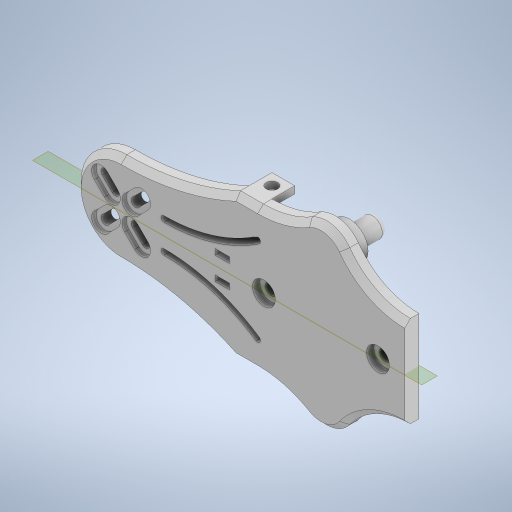
# Autodesk Inventor part: BLDC_Arm_2
Saved by Autodesk Inventor 2024 (Build 280153000, 153)
## iProperties
Created: 2024-04-12
Part Number: BLDC_Arm_2
Material: Generic
Document SubType Name: Modeling
Designer: CJ110
Density: 1 g/cm^3
Appearance: Default
Author: CJ110
Autodesk Inventor part; units mm, degrees
ref_plane "YZ Plane" through (0, 0, 0) normal (1, 0, 0) x (0, 1, 0)
ref_plane "XZ Plane" through (0, 0, 0) normal (0, 1, 0) x (-1, 0, 0)
ref_plane "XY Plane" through (0, 0, 0) normal (0, 0, 1) x (1, 0, 0)
sketch "Sketch1" plane through (0, 0, 0) normal (0, 0, 1) x (1, 0, 0)
  arc A0 (0, 16) -> (0, -16) centre (0, 0) ccw
  line L0 (0, 16) -> (99.4033, 16)
  line L1 (99.4033, 16) -> (99.4033, -16)
  line L2 (99.4033, -16) -> (0, -16)
  line L3 (0, -16) -> (0, 16) construction
  line L4 (39.8634, 25) -> (99.4033, 25)
  line L5 (99.4033, 25) -> (99.4033, -25)
  line L6 (99.4033, -25) -> (39.8634, -25)
  line L7 (39.8634, -25) -> (39.8634, 25)
  arc A1 (39.8634, -25) -> (0, -16) centre (0, -108.7828) ccw
  arc A2 (0, 16) -> (39.8634, 25) centre (0, 108.7828) ccw
  circle A3 centre (50.0625, 0) radius 2
  circle A4 centre (90.0625, 0) radius 2
  line L8 (-16, 0) -> (99.4033, 0) construction
  line L9 (-7.0711, 7.0711) -> (-3.5356, 3.5356) construction
  line L10 (-8.1318, 6.0104) -> (-4.5962, 2.4749)
  line L11 (-2.4749, 4.5962) -> (-6.0104, 8.1318)
  arc A5 (-6.0104, 8.1318) -> (-8.1318, 6.0104) centre (-7.0711, 7.0711) ccw
  arc A6 (-4.5962, 2.4749) -> (-2.4749, 4.5962) centre (-3.5356, 3.5356) ccw
  line L12 (0, 0) -> (-8.1318, 8.1318) construction
  arc A7 (-2.4749, -4.5962) -> (-4.5962, -2.4749) centre (-3.5356, -3.5356) ccw
  line L13 (-4.5962, -2.4749) -> (-8.1318, -6.0104)
  arc A8 (-8.1318, -6.0104) -> (-6.0104, -8.1318) centre (-7.0711, -7.0711) ccw
  line L14 (-6.0104, -8.1318) -> (-2.4749, -4.5962)
  arc A9 (4.5962, -2.4749) -> (2.4749, -4.5962) centre (3.5356, -3.5356) ccw
  line L15 (2.4749, -4.5962) -> (6.0104, -8.1318)
  arc A10 (6.0104, -8.1318) -> (8.1318, -6.0104) centre (7.0711, -7.0711) ccw
  line L16 (8.1318, -6.0104) -> (4.5962, -2.4749)
  arc A11 (2.4749, 4.5962) -> (4.5962, 2.4749) centre (3.5356, 3.5356) ccw
  line L17 (4.5962, 2.4749) -> (8.1318, 6.0104)
  arc A12 (8.1318, 6.0104) -> (6.0104, 8.1318) centre (7.0711, 7.0711) ccw
  line L18 (6.0104, 8.1318) -> (2.4749, 4.5962)
  point P0 (39.8634, 0)
  point P1 (99.4033, -16)
  point P2 (99.4033, 16)
  point P3 (-5.3033, 5.3033)
  point P4 (-2.4749, 2.4749)
  point P5 (-2.4749, -2.4749)
  point P6 (-8.1318, -8.1318)
  point P7 (2.4749, -2.4749)
  point P8 (8.1318, -8.1318)
  point P9 (2.4749, 2.4749)
  point P10 (8.1318, 8.1318)
  dimension "d3" = 50
  dimension "d4" = 59.5399
  dimension "d12" = 4
  dimension "d13" = 40
  dimension "d15" = 9.3408
  dimension "d44" = 16
  dimension "d45" = 99.4033
  dimension "d46" = 3
  dimension "d47" = 8
  dimension "d48" = 45
  dimension "d49" = 2.4749
  dimension "d52" = 360
  constraints: 40 end point, 25 point on circle, 13 centre point, 7 tangent, 5 parallel, 4 midpoint, 3 horizontal, 2 collinear, 2 perpendicular, 2 point on line, 1 coincident, 1 equal radius, 1 horizontal alignment, 49 other
  measures "d3" distance between parallel lines of L6 L4
  measures "d4" distance between parallel lines of L5 L7
  measures "d12" diameter of A4
  measures "d13" distance of A3.centre A4.centre
  measures "d15" distance from line of L1 A4.centre
  measures "d44" radius of A0
  measures "d45" distance from line of point (0, 0) L5
  measures "d46" distance between parallel lines of L10 L11
  measures "d47" distance of point (-2.475, 2.475) L12.end
  measures "d48" angle of L8 L12
  measures "d49" distance from line of L8 point (-2.475, 2.475)
extrude "Extrusion1" add sketch "Sketch1" along normal blind 5
ref_plane "Work Plane1" through (39.8634, 0, 0) normal (0, -1, 0) x (1, 0, 0)
sketch "Sketch4" plane through (0, 0, 5) normal (0, 0, 1) x (1, 0, 0)
  arc A0 (15, 6) -> (47.3064, 15.8305) centre (15, 64.0002) ccw
  arc A1 (15, 4) -> (48.4204, 14.1695) centre (15, 64.0002) ccw
  circle A2 centre (47.8634, 15) radius 1
  circle A3 centre (15, 5) radius 1
  arc A4 (0, 16) -> (39.8634, 25) centre (0, 108.7828) ccw projected
  line L0 (99.4033, 25) -> (39.8634, 25) projected
  line L1 (122.484, 0) -> (-39.0807, 0) projected
  line L2 (15, 4) -> (47.8634, 4) construction
  point P0 (0, 0)
  dimension "d16" = 2
  dimension "d17" = 10
  dimension "d18" = 8
  dimension "d19" = 15
  dimension "d20" = 5
  constraints: 8 point on circle, 5 tangent, 4 centre point, 2 end point, 1 concentric, 1 equal radius, 1 horizontal, 1 vertical alignment
  measures "d16" diameter of A2
  measures "d17" distance from line of L0 A2.centre
  measures "d18" horizontal distance of L0.end A2.centre
  measures "d19" horizontal distance of point (0, 0) A3.centre
  measures "d20" distance from line of L1 A3.centre
extrude "Extrusion3" cut sketch "Sketch4" against normal through all
mirror "Mirror1" about plane through (39.8634, 0, 0) normal (0, -1, 0) of "Extrusion3"
sketch "Sketch5" plane through (0, 0, 0) normal (0, 0, -1) x (-1, 0, 0)
  arc A0 (-15, -4) -> (-48.4204, -14.1695) centre (-15, -64.0002) ccw projected
  arc A1 (-15, -6) -> (-15, -4) centre (-15, -5) ccw projected
  arc A2 (-15, -6) -> (-47.3064, -15.8305) centre (-15, -64.0002) ccw projected
  arc A3 (-48.4204, -14.1695) -> (-47.3064, -15.8305) centre (-47.8634, -15) ccw projected
  arc A4 (-47.3064, 15.8305) -> (-15, 6) centre (-15, 64.0002) ccw projected
  arc A5 (-15, 4) -> (-15, 6) centre (-15, 5) ccw projected
  arc A6 (-48.4204, 14.1695) -> (-15, 4) centre (-15, 64.0002) ccw projected
  arc A7 (-47.3064, 15.8305) -> (-48.4204, 14.1695) centre (-47.8634, 15) ccw projected
  arc A8 (0, -16) -> (0, 16) centre (0, 0) ccw projected
  arc A9 (-39.8634, 25) -> (0, 16) centre (0, 108.7828) ccw projected
  line L0 (-99.4033, 25) -> (-39.8634, 25) projected
  line L1 (-99.4033, -25) -> (-99.4033, 25) projected
  line L2 (-39.8634, -25) -> (-99.4033, -25) projected
  arc A10 (0, -16) -> (-39.8634, -25) centre (0, -108.7828) ccw projected
  circle A11 centre (-50.0625, 0) radius 2 projected
  circle A12 centre (-90.0625, 0) radius 2 projected
  line L3 (-39.8634, 25) -> (-47.8634, 25)
  line L4 (-47.8634, 25) -> (-47.8634, 22.5)
  line L5 (-47.8634, 22.5) -> (-39.8634, 22.5)
  line L6 (-39.8634, 22.5) -> (-39.8634, 25)
  dimension "d23" = 8
  dimension "d24" = 2.5
  constraints: 8 end point, 2 parallel, 1 horizontal, 1 perpendicular
  measures "d23" distance of L4.end L5.end
  measures "d24" distance of L3.end L4.end
extrude "Extrusion4" add sketch "Sketch5" along normal blind 8 contours L6 L5 L4 L0
sketch "Sketch6" plane through (39.8634, 25, 5) normal (0, 1, 0) x (1, 0, 0)
  line L0 (59.5399, 5) -> (8, 5) projected
  line L1 (8, 5) -> (8, 13) projected
  line L2 (0, 13) -> (8, 13) projected
  line L3 (0, 5) -> (0, 13) projected
  line L4 (0, 5) -> (0, 0) projected
  line L5 (59.5399, 0) -> (0, 0) projected
  line L6 (59.5399, 5) -> (59.5399, 0) projected
  circle A0 centre (4, 9) radius 2
  line L7 (4, 13) -> (4, 9) construction
  point P0 (-39.8634, 5)
  dimension "d27" = 4
  dimension "d28" = 4
  constraints: 2 end point, 1 centre point, 1 midpoint, 1 vertical
  measures "d27" distance from line of L2 L7.end
  measures "d28" diameter of A0
extrude "Extrusion5" cut sketch "Sketch6" against normal up to next contours A0
mirror "Mirror2" about plane through (39.8634, 0, 0) normal (0, -1, 0) of "Extrusion4", "Extrusion5"
sketch "Sketch7" plane through (0, 0, 0) normal (0, 0, -1) x (-1, 0, 0)
  circle A0 centre (-90.0625, 0) radius 2 projected
  circle A1 centre (-50.0625, 0) radius 2 projected
  arc A2 (-47.3064, 15.8305) -> (-15, 6) centre (-15, 64.0002) ccw projected
  arc A3 (-15, 4) -> (-15, 6) centre (-15, 5) ccw projected
  arc A4 (-48.4204, 14.1695) -> (-15, 4) centre (-15, 64.0002) ccw projected
  arc A5 (-47.3064, 15.8305) -> (-48.4204, 14.1695) centre (-47.8634, 15) ccw projected
  arc A6 (-15, -4) -> (-48.4204, -14.1695) centre (-15, -64.0002) ccw projected
  arc A7 (-15, -6) -> (-15, -4) centre (-15, -5) ccw projected
  arc A8 (-15, -6) -> (-47.3064, -15.8305) centre (-15, -64.0002) ccw projected
  arc A9 (-48.4204, -14.1695) -> (-47.3064, -15.8305) centre (-47.8634, -15) ccw projected
  line L0 (-47.8634, -25) -> (-47.8634, -22.5) projected
  line L1 (-47.8634, -22.5) -> (-39.8634, -22.5) projected
  line L2 (-39.8634, -22.5) -> (-39.8634, -25) projected
  arc A10 (0, -16) -> (-39.8634, -25) centre (0, -108.7828) ccw projected
  arc A11 (0, -16) -> (0, 16) centre (0, 0) ccw projected
  arc A12 (-39.8634, 25) -> (0, 16) centre (0, 108.7828) ccw projected
  line L3 (-39.8634, 25) -> (-39.8634, 22.5) projected
  line L4 (-39.8634, 22.5) -> (-47.8634, 22.5) projected
  line L5 (-47.8634, 22.5) -> (-47.8634, 25) projected
  line L6 (-99.4033, 25) -> (-47.8634, 25) projected
  line L7 (-99.4033, -25) -> (-99.4033, 25) projected
  line L8 (-47.8634, -25) -> (-99.4033, -25) projected
  circle A13 centre (-70.0625, 21) radius 10
  arc A14 (-65.0249, 29.6384) -> (-47.8634, 25) centre (-47.8634, 59.0667) ccw
  line L9 (-99.4033, 25) -> (-47.8634, 25) projected
  line L10 (39.0807, 0) -> (-122.484, 0) projected
  line L11 (-70.0625, -25) -> (-70.0625, 21) construction
  line L12 (-90.0625, 0) -> (-50.0625, 0) construction
  line L13 (0, 16) -> (-99.4033, 16) construction
  arc A15 (-99.4033, 16) -> (-78.1686, 26.8559) centre (-99.4033, 42.1961) ccw
  point P0 (-92.2616, 25)
  point P1 (-75.1001, 29.6384)
  point P2 (-70.0625, 0)
  point P3 (-60.8973, 25)
  point P4 (-79.2277, 25)
  point P5 (-79.6415, 25)
  dimension "d31" = 20
  dimension "d32" = 21
  constraints: 7 point on circle, 6 end point, 5 tangent, 4 point on line, 3 centre point, 2 perpendicular, 1 coincident, 1 collinear, 1 midpoint, 1 vertical
  measures "d31" diameter of A13
  measures "d32" distance from line of L10 A13.centre
extrude "Extrusion6" add sketch "Sketch7" against normal up to surface (5 mm away) contours A15 A13 L6 | A13 L6 | A13 A14 L6 picked at (-69.5865, 27.6164)
sketch "Sketch8" plane through (0, 0, 0) normal (0, 0, -1) x (-1, 0, 0)
  circle A0 centre (-90.0625, 0) radius 2 projected
  circle A1 centre (-50.0625, 0) radius 2 projected
  arc A2 (-47.3064, 15.8305) -> (-15, 6) centre (-15, 64.0002) ccw projected
  arc A3 (-15, 4) -> (-15, 6) centre (-15, 5) ccw projected
  arc A4 (-48.4204, 14.1695) -> (-15, 4) centre (-15, 64.0002) ccw projected
  arc A5 (-47.3064, 15.8305) -> (-48.4204, 14.1695) centre (-47.8634, 15) ccw projected
  arc A6 (-15, -4) -> (-48.4204, -14.1695) centre (-15, -64.0002) ccw projected
  arc A7 (-15, -6) -> (-15, -4) centre (-15, -5) ccw projected
  arc A8 (-15, -6) -> (-47.3064, -15.8305) centre (-15, -64.0002) ccw projected
  arc A9 (-48.4204, -14.1695) -> (-47.3064, -15.8305) centre (-47.8634, -15) ccw projected
  line L0 (-47.8634, -25) -> (-47.8634, -22.5) projected
  line L1 (-47.8634, -22.5) -> (-39.8634, -22.5) projected
  line L2 (-39.8634, -22.5) -> (-39.8634, -25) projected
  arc A10 (0, -16) -> (-39.8634, -25) centre (0, -108.7828) ccw projected
  arc A11 (0, -16) -> (0, 16) centre (0, 0) ccw projected
  arc A12 (-39.8634, 25) -> (0, 16) centre (0, 108.7828) ccw projected
  line L3 (-39.8634, 25) -> (-39.8634, 22.5) projected
  line L4 (-39.8634, 22.5) -> (-47.8634, 22.5) projected
  line L5 (-47.8634, 22.5) -> (-47.8634, 25) projected
  arc A13 (-65.0249, 29.6384) -> (-47.8634, 25) centre (-47.8634, 59.0667) ccw projected
  arc A14 (-65.0249, 29.6384) -> (-78.1686, 26.8559) centre (-70.0625, 21) ccw projected
  line L6 (-99.4033, 25) -> (-79.6415, 25) projected
  line L7 (-99.4033, -25) -> (-99.4033, 25) projected
  line L8 (-47.8634, -25) -> (-99.4033, -25) projected
  circle A15 centre (-70.0625, 21) radius 6.5
  arc A16 (-79.6415, 25) -> (-78.1686, 26.8559) centre (-99.4033, 42.1961) ccw projected
  dimension "d35" = 13
  constraints: 1 centre point, 1 coincident
  measures "d35" diameter of A15
extrude "Extrusion7" add sketch "Sketch8" along normal blind 5 contours A15
sketch "Sketch9" plane through (70.0625, 21, -5) normal (0, 0, -1) x (-1, 0, 0)
  circle A0 centre (0, 0) radius 3.5
  circle A1 centre (0, 0) radius 6.5 projected
  point P0 (70.0625, -21)
  dimension "d38" = 7
  constraints: 1 centre point, 1 coincident
  measures "d38" diameter of A0
extrude "Extrusion8" add sketch "Sketch9" along normal blind 10 contours A0
fillet "Fillet1" radius 2 1 edges at (73.5625, 21, -15)
extrude "Extrusion9" cut sketch "Sketch7" against normal through all contours L7 L6 A15
mirror "Mirror3" about plane through (39.8634, 0, 0) normal (0, -1, 0) of "Extrusion6", "Extrusion7", "Extrusion8", "Fillet1", "Extrusion9"
sketch "Sketch11" plane through (0, 0, 0) normal (0, 0, -1) x (-1, 0, 0)
  line L0 (-45, 3) -> (-10, 3)
  line L1 (-10, 3) -> (-10, -3)
  line L2 (-10, -3) -> (-45, -3)
  line L3 (-45, -3) -> (-45, 3)
  line L4 (39.0807, 0) -> (-122.484, 0) projected
  point P0 (0, 0)
  point P1 (-10, 0)
  dimension "d54" = 6
  dimension "d55" = 10
  dimension "d56" = 35
  constraints: 8 end point, 2 parallel, 1 horizontal, 1 midpoint, 1 perpendicular, 1 point on line
  measures "d54" distance between parallel lines of L2 L0
  measures "d55" distance from line of point (0, 0) L1
  measures "d56" distance of L1.end L2.end
extrude "Extrusion10" cut sketch "Sketch11" against normal blind 2
sketch "Sketch12" plane through (39.8634, 0, 0) normal (0, -1, 0) x (1, 0, 0)
  line L0 (-29.8634, 0) -> (5.1366, 0) projected
  line L1 (5.1366, 0) -> (-29.8634, 0) projected
  line L2 (59.5399, 0) -> (38.3052, 0) projected
  line L3 (25.1615, 0) -> (38.3052, 0) projected
  line L4 (8, 0) -> (25.1615, 0) projected
  line L5 (8, 0) -> (0, 0) projected
  line L6 (-39.8634, 0) -> (0, 0) projected
  line L7 (-39.8634, 0) -> (-39.8634, 0) projected
  line L8 (0, 0) -> (-39.8634, 0) projected
  line L9 (0, 0) -> (8, 0) projected
  line L10 (8, 0) -> (25.1615, 0) projected
  line L11 (25.1615, 0) -> (38.3052, 0) projected
  line L12 (38.3052, 0) -> (59.5399, 0) projected
  line L13 (36.6991, 0) -> (23.6991, 0) projected
  line L14 (36.6991, 0) -> (23.6991, 0) projected
  line L15 (-37.3885, 0) -> (-33.853, 0) projected
  line L16 (-35.2672, 0) -> (-37.3885, 0) projected
  line L17 (-31.7316, 0) -> (-35.2672, 0) projected
  line L18 (-33.853, 0) -> (-31.7316, 0) projected
  line L19 (-35.2672, 0) -> (-31.7316, 0) projected
  line L20 (-37.3885, 0) -> (-35.2672, 0) projected
  line L21 (-33.853, 0) -> (-37.3885, 0) projected
  line L22 (-31.7316, 0) -> (-33.853, 0) projected
  line L23 (-42.3383, 0) -> (-45.8738, 0) projected
  line L24 (-44.4596, 0) -> (-42.3383, 0) projected
  line L25 (-47.9952, 0) -> (-44.4596, 0) projected
  line L26 (-45.8738, 0) -> (-47.9952, 0) projected
  line L27 (-47.9952, 0) -> (-45.8738, 0) projected
  line L28 (-44.4596, 0) -> (-47.9952, 0) projected
  line L29 (-42.3383, 0) -> (-44.4596, 0) projected
  line L30 (-45.8738, 0) -> (-42.3383, 0) projected
  line L31 (48.1991, 0) -> (52.1991, 0) projected
  line L32 (8.1991, 0) -> (12.1991, 0) projected
  line L33 (7.443, 0) -> (-24.8634, 0) projected
  line L34 (-24.8634, 0) -> (-24.8634, 0) projected
  line L35 (-24.8634, 0) -> (8.557, 0) projected
  line L36 (8.557, 0) -> (7.443, 0) projected
  line L37 (8.557, 0) -> (-24.8634, 0) projected
  line L38 (-24.8634, 0) -> (-24.8634, 0) projected
  line L39 (-24.8634, 0) -> (7.443, 0) projected
  line L40 (7.443, 0) -> (8.557, 0) projected
  arc A0 (-36.8634, 0) -> (-39.8634, 3) centre (-39.8634, 0) ccw
  line L41 (-39.8634, 0) -> (-39.8634, 3)
  dimension "d59" = 3
  constraints: 2 end point, 2 point on circle, 1 centre point, 1 coincident, 1 perpendicular, 1 point on line
  measures "d59" distance of point (-39.863, 0) A0.start
revolve "Revolution1" cut sketch "Sketch12" angle 360 about axis through (0, 0, 0) along (0, 0, 1)
sketch "Sketch13" plane through (0, 0, 0) normal (0, 0, -1) x (-1, 0, 0)
  circle A0 centre (0, 0) radius 3 projected
  line L0 (-10, -3) -> (-45, -3) projected
  line L1 (-45, -3) -> (-45, 3) projected
  line L2 (-45, 3) -> (-10, 3) projected
  line L3 (-10, 3) -> (-10, -3) projected
  arc A1 (-78.1686, -26.8559) -> (-99.4033, -16) centre (-99.4033, -42.1961) ccw projected
  arc A2 (-78.1686, -26.8559) -> (-65.0249, -29.6384) centre (-70.0625, -21) ccw projected
  arc A3 (-47.8634, -25) -> (-65.0249, -29.6384) centre (-47.8634, -59.0667) ccw projected
  line L4 (-47.8634, -25) -> (-47.8634, -22.5) projected
  line L5 (-47.8634, -22.5) -> (-39.8634, -22.5) projected
  line L6 (-39.8634, -22.5) -> (-39.8634, -25) projected
  arc A4 (0, -16) -> (-39.8634, -25) centre (0, -108.7828) ccw projected
  arc A5 (0, -16) -> (0, 16) centre (0, 0) ccw projected
  arc A6 (-39.8634, 25) -> (0, 16) centre (0, 108.7828) ccw projected
  line L7 (-39.8634, 25) -> (-39.8634, 22.5) projected
  line L8 (-39.8634, 22.5) -> (-47.8634, 22.5) projected
  line L9 (-47.8634, 22.5) -> (-47.8634, 25) projected
  arc A7 (-65.0249, 29.6384) -> (-47.8634, 25) centre (-47.8634, 59.0667) ccw projected
  arc A8 (-65.0249, 29.6384) -> (-78.1686, 26.8559) centre (-70.0625, 21) ccw projected
  arc A9 (-99.4033, 16) -> (-78.1686, 26.8559) centre (-99.4033, 42.1961) ccw projected
  line L10 (-99.4033, -16) -> (-99.4033, 16) projected
  circle A10 centre (-70.0625, -21) radius 6.5 projected
  circle A11 centre (-70.0625, 21) radius 6.5 projected
  line L11 (-2.4749, 4.5962) -> (-6.0104, 8.1318) projected
  arc A12 (-4.5962, 2.4749) -> (-2.4749, 4.5962) centre (-3.5356, 3.5356) ccw projected
  line L12 (-8.1318, 6.0104) -> (-4.5962, 2.4749) projected
  arc A13 (-6.0104, 8.1318) -> (-8.1318, 6.0104) centre (-7.0711, 7.0711) ccw projected
  line L13 (-4.5962, -2.4749) -> (-8.1318, -6.0104) projected
  arc A14 (-2.4749, -4.5962) -> (-4.5962, -2.4749) centre (-3.5356, -3.5356) ccw projected
  line L14 (-6.0104, -8.1318) -> (-2.4749, -4.5962) projected
  arc A15 (-8.1318, -6.0104) -> (-6.0104, -8.1318) centre (-7.0711, -7.0711) ccw projected
  line L15 (2.4749, -4.5962) -> (6.0104, -8.1318) projected
  arc A16 (4.5962, -2.4749) -> (2.4749, -4.5962) centre (3.5356, -3.5356) ccw projected
  line L16 (8.1318, -6.0104) -> (4.5962, -2.4749) projected
  arc A17 (6.0104, -8.1318) -> (8.1318, -6.0104) centre (7.0711, -7.0711) ccw projected
  arc A18 (8.1318, 6.0104) -> (6.0104, 8.1318) centre (7.0711, 7.0711) ccw projected
  line L17 (4.5962, 2.4749) -> (8.1318, 6.0104) projected
  arc A19 (2.4749, 4.5962) -> (4.5962, 2.4749) centre (3.5356, 3.5356) ccw projected
  line L18 (6.0104, 8.1318) -> (2.4749, 4.5962) projected
  circle A20 centre (-90.0625, 0) radius 2 projected
  circle A21 centre (-50.0625, 0) radius 2 projected
  arc A22 (-47.3064, 15.8305) -> (-15, 6) centre (-15, 64.0002) ccw projected
  arc A23 (-15, 4) -> (-15, 6) centre (-15, 5) ccw projected
  arc A24 (-48.4204, 14.1695) -> (-15, 4) centre (-15, 64.0002) ccw projected
  arc A25 (-47.3064, 15.8305) -> (-48.4204, 14.1695) centre (-47.8634, 15) ccw projected
  arc A26 (-15, -4) -> (-48.4204, -14.1695) centre (-15, -64.0002) ccw projected
  arc A27 (-15, -6) -> (-15, -4) centre (-15, -5) ccw projected
  arc A28 (-15, -6) -> (-47.3064, -15.8305) centre (-15, -64.0002) ccw projected
  arc A29 (-48.4204, -14.1695) -> (-47.3064, -15.8305) centre (-47.8634, -15) ccw projected
  line L19 (-38, 3) -> (-33, 3)
  line L20 (-33, 3) -> (-33, 5)
  line L21 (-33, 5) -> (-38, 5)
  line L22 (-38, 5) -> (-38, 3)
  dimension "d61" = 2
  dimension "d62" = 5
  dimension "d63" = 7
  constraints: 8 end point, 2 parallel, 1 horizontal, 1 perpendicular, 1 point on line
  measures "d61" distance between parallel lines of L2 L21
  measures "d62" distance of L20.end L21.end
  measures "d63" distance between parallel lines of L1 L22
extrude "Extrusion11" cut sketch "Sketch13" against normal through all contours L2 L22 L21 L20
mirror "Mirror4" about plane through (39.8634, 0, 0) normal (0, -1, 0) of "Extrusion11"
sketch "Sketch14" plane through (0, 0, 5) normal (0, 0, 1) x (1, 0, 0)
  line L0 (38, -5) -> (33, -5) projected
  line L1 (33, -5) -> (33, -3) projected
  line L2 (33, -3) -> (38, -3) projected
  line L3 (38, -3) -> (38, -5) projected
  line L4 (38, 3) -> (33, 3) projected
  line L5 (33, 3) -> (33, 5) projected
  line L6 (33, 5) -> (38, 5) projected
  line L7 (38, 5) -> (38, 3) projected
  arc A0 (48.4204, -14.1695) -> (15, -4) centre (15, -64.0002) ccw projected
  arc A1 (47.3064, -15.8305) -> (48.4204, -14.1695) centre (47.8634, -15) ccw projected
  arc A2 (47.3064, -15.8305) -> (15, -6) centre (15, -64.0002) ccw projected
  arc A3 (15, -4) -> (15, -6) centre (15, -5) ccw projected
  arc A4 (15, 6) -> (47.3064, 15.8305) centre (15, 64.0002) ccw projected
  arc A5 (48.4204, 14.1695) -> (47.3064, 15.8305) centre (47.8634, 15) ccw projected
  arc A6 (15, 4) -> (48.4204, 14.1695) centre (15, 64.0002) ccw projected
  arc A7 (15, 6) -> (15, 4) centre (15, 5) ccw projected
  arc A8 (99.4033, -16) -> (78.1686, -26.8559) centre (99.4033, -42.1961) ccw projected
  line L8 (99.4033, -16) -> (99.4033, 16) projected
  arc A9 (78.1686, 26.8559) -> (99.4033, 16) centre (99.4033, 42.1961) ccw projected
  line L9 (47.8634, 25) -> (39.8634, 25) projected
  arc A10 (78.1686, 26.8559) -> (65.0249, 29.6384) centre (70.0625, 21) ccw projected
  arc A11 (47.8634, 25) -> (65.0249, 29.6384) centre (47.8634, 59.0667) ccw projected
  arc A12 (0, 16) -> (39.8634, 25) centre (0, 108.7828) ccw projected
  arc A13 (0, 16) -> (0, -16) centre (0, 0) ccw projected
  arc A14 (39.8634, -25) -> (0, -16) centre (0, -108.7828) ccw projected
  line L10 (39.8634, -25) -> (47.8634, -25) projected
  arc A15 (65.0249, -29.6384) -> (47.8634, -25) centre (47.8634, -59.0667) ccw projected
  arc A16 (65.0249, -29.6384) -> (78.1686, -26.8559) centre (70.0625, -21) ccw projected
  circle A17 centre (50.0625, 0) radius 2 projected
  circle A18 centre (90.0625, 0) radius 2 projected
  arc A19 (-6.0104, 8.1318) -> (-8.1318, 6.0104) centre (-7.0711, 7.0711) ccw projected
  line L11 (-6.0104, 8.1318) -> (-2.4749, 4.5962) projected
  arc A20 (-4.5962, 2.4749) -> (-2.4749, 4.5962) centre (-3.5356, 3.5356) ccw projected
  line L12 (-4.5962, 2.4749) -> (-8.1318, 6.0104) projected
  line L13 (-2.4749, -4.5962) -> (-6.0104, -8.1318) projected
  arc A21 (-8.1318, -6.0104) -> (-6.0104, -8.1318) centre (-7.0711, -7.0711) ccw projected
  line L14 (-8.1318, -6.0104) -> (-4.5962, -2.4749) projected
  arc A22 (-2.4749, -4.5962) -> (-4.5962, -2.4749) centre (-3.5356, -3.5356) ccw projected
  line L15 (4.5962, -2.4749) -> (8.1318, -6.0104) projected
  arc A23 (6.0104, -8.1318) -> (8.1318, -6.0104) centre (7.0711, -7.0711) ccw projected
  line L16 (6.0104, -8.1318) -> (2.4749, -4.5962) projected
  arc A24 (4.5962, -2.4749) -> (2.4749, -4.5962) centre (3.5356, -3.5356) ccw projected
  line L17 (2.4749, 4.5962) -> (6.0104, 8.1318) projected
  arc A25 (8.1318, 6.0104) -> (6.0104, 8.1318) centre (7.0711, 7.0711) ccw projected
  line L18 (8.1318, 6.0104) -> (4.5962, 2.4749) projected
  arc A26 (2.4749, 4.5962) -> (4.5962, 2.4749) centre (3.5356, 3.5356) ccw projected
  line L19 (-1.2375, 5.8337) -> (-4.773, 9.3692)
  arc A27 (-4.773, 9.3692) -> (-9.3692, 4.773) centre (-7.0711, 7.0711) ccw
  line L20 (-9.3692, 4.773) -> (-5.8337, 1.2375)
  arc A28 (-5.8337, 1.2375) -> (-1.2375, 5.8337) centre (-3.5356, 3.5356) ccw
  line L21 (4.773, 9.3692) -> (1.2375, 5.8337)
  arc A29 (1.2375, 5.8337) -> (5.8337, 1.2375) centre (3.5356, 3.5356) ccw
  line L22 (5.8337, 1.2375) -> (9.3692, 4.773)
  arc A30 (9.3692, 4.773) -> (4.773, 9.3692) centre (7.0711, 7.0711) ccw
  line L23 (9.3692, -4.773) -> (5.8337, -1.2375)
  arc A31 (5.8337, -1.2375) -> (1.2375, -5.8337) centre (3.5356, -3.5356) ccw
  line L24 (1.2375, -5.8337) -> (4.773, -9.3692)
  arc A32 (4.773, -9.3692) -> (9.3692, -4.773) centre (7.0711, -7.0711) ccw
  line L25 (-4.773, -9.3692) -> (-1.2375, -5.8337)
  arc A33 (-1.2375, -5.8337) -> (-5.8337, -1.2375) centre (-3.5356, -3.5356) ccw
  line L26 (-5.8337, -1.2375) -> (-9.3692, -4.773)
  arc A34 (-9.3692, -4.773) -> (-4.773, -9.3692) centre (-7.0711, -7.0711) ccw
  dimension "d66" = 1.75
  constraints: 16 end point, 16 point on circle, 8 centre point, 3 equal radius, 12 other
  measures "d66" distance between parallel lines of L11 L19
extrude "Extrusion12" cut sketch "Sketch14" against normal blind 1.5 contours A28 L20 A27 L19 | A30 L22 A29 L21 | A32 L24 A31 L23 | A34 L26 A33 L25
sketch "Sketch15" plane through (0, 0, 5) normal (0, 0, 1) x (1, 0, 0)
  line L0 (4.773, -9.3692) -> (1.2375, -5.8337) projected
  arc A0 (5.8337, -1.2375) -> (1.2375, -5.8337) centre (3.5356, -3.5356) ccw projected
  line L1 (5.8337, -1.2375) -> (9.3692, -4.773) projected
  arc A1 (4.773, -9.3692) -> (9.3692, -4.773) centre (7.0711, -7.0711) ccw projected
  line L2 (9.3692, 4.773) -> (5.8337, 1.2375) projected
  arc A2 (1.2375, 5.8337) -> (5.8337, 1.2375) centre (3.5356, 3.5356) ccw projected
  line L3 (1.2375, 5.8337) -> (4.773, 9.3692) projected
  arc A3 (9.3692, 4.773) -> (4.773, 9.3692) centre (7.0711, 7.0711) ccw projected
  line L4 (-9.3692, -4.773) -> (-5.8337, -1.2375) projected
  arc A4 (-1.2375, -5.8337) -> (-5.8337, -1.2375) centre (-3.5356, -3.5356) ccw projected
  line L5 (-1.2375, -5.8337) -> (-4.773, -9.3692) projected
  arc A5 (-9.3692, -4.773) -> (-4.773, -9.3692) centre (-7.0711, -7.0711) ccw projected
  line L6 (-5.8337, 1.2375) -> (-9.3692, 4.773) projected
  arc A6 (-4.773, 9.3692) -> (-9.3692, 4.773) centre (-7.0711, 7.0711) ccw projected
  line L7 (-4.773, 9.3692) -> (-1.2375, 5.8337) projected
  arc A7 (-5.8337, 1.2375) -> (-1.2375, 5.8337) centre (-3.5356, 3.5356) ccw projected
  line L8 (38, -5) -> (33, -5) projected
  line L9 (33, -5) -> (33, -3) projected
  line L10 (33, -3) -> (38, -3) projected
  line L11 (38, -3) -> (38, -5) projected
  line L12 (38, 3) -> (33, 3) projected
  line L13 (33, 3) -> (33, 5) projected
  line L14 (33, 5) -> (38, 5) projected
  line L15 (38, 5) -> (38, 3) projected
  arc A8 (48.4204, -14.1695) -> (15, -4) centre (15, -64.0002) ccw projected
  arc A9 (47.3064, -15.8305) -> (48.4204, -14.1695) centre (47.8634, -15) ccw projected
  arc A10 (47.3064, -15.8305) -> (15, -6) centre (15, -64.0002) ccw projected
  arc A11 (15, -4) -> (15, -6) centre (15, -5) ccw projected
  arc A12 (15, 6) -> (47.3064, 15.8305) centre (15, 64.0002) ccw projected
  arc A13 (48.4204, 14.1695) -> (47.3064, 15.8305) centre (47.8634, 15) ccw projected
  arc A14 (15, 4) -> (48.4204, 14.1695) centre (15, 64.0002) ccw projected
  arc A15 (15, 6) -> (15, 4) centre (15, 5) ccw projected
  arc A16 (99.4033, -16) -> (78.1686, -26.8559) centre (99.4033, -42.1961) ccw projected
  line L16 (99.4033, -16) -> (99.4033, 16) projected
  arc A17 (78.1686, 26.8559) -> (99.4033, 16) centre (99.4033, 42.1961) ccw projected
  line L17 (47.8634, 25) -> (39.8634, 25) projected
  arc A18 (78.1686, 26.8559) -> (65.0249, 29.6384) centre (70.0625, 21) ccw projected
  arc A19 (47.8634, 25) -> (65.0249, 29.6384) centre (47.8634, 59.0667) ccw projected
  arc A20 (0, 16) -> (39.8634, 25) centre (0, 108.7828) ccw projected
  arc A21 (0, 16) -> (0, -16) centre (0, 0) ccw projected
  arc A22 (39.8634, -25) -> (0, -16) centre (0, -108.7828) ccw projected
  line L18 (39.8634, -25) -> (47.8634, -25) projected
  arc A23 (65.0249, -29.6384) -> (47.8634, -25) centre (47.8634, -59.0667) ccw projected
  arc A24 (65.0249, -29.6384) -> (78.1686, -26.8559) centre (70.0625, -21) ccw projected
  circle A25 centre (50.0625, 0) radius 2 projected
  circle A26 centre (90.0625, 0) radius 2 projected
  circle A27 centre (50.0625, 0) radius 4
  circle A28 centre (90.0625, 0) radius 4
  dimension "d69" = 8
  constraints: 2 centre point, 2 coincident, 1 equal radius
  measures "d69" diameter of A28
extrude "Extrusion13" cut sketch "Sketch15" against normal blind 2.5 contours A27 | A28
fillet "Fillet2" radius 2 4 edges at (41.5, 3, 2) (41.5, -3, 2) (21.5, 3, 2) (21.5, -3, 2)
chamfer "Chamfer1" distance 2 angle 45 11 edges at (20.4334, 18.278, 5) (-16, 0, 5) (20.4334, -18.278, 5) (43.8634, 25, 5) (56.752, 26.18, 5) (72.1336, 30.7832, 5) (87.4789, 18.8713, 5) (56.752, -26.18, 5) (72.1336, -30.7832, 5) (87.4789, -18.8713, 5) (43.8634, -25, 5)
body "Solid1"
